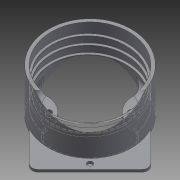
# Autodesk Inventor part: DiffuserCoupler
Saved by Autodesk Inventor 2014 SP2 (Build 180246200, 246)
## iProperties
Created: 2014-02-09
Part Number: DiffuserCoupler
Material: Generic
Document SubType Name: Modeling
Designer: jkao
Density: 1 g/cm^3
Appearance: Default
Author: jkao
Autodesk Inventor part; units mm, degrees
ref_plane "YZ Plane" through (0, 0, 0) normal (1, 0, 0) x (0, 1, 0)
ref_plane "XZ Plane" through (0, 0, 0) normal (0, 1, 0) x (-1, 0, 0)
ref_plane "XY Plane" through (0, 0, 0) normal (0, 0, 1) x (1, 0, 0)
sketch "Collar Profile" plane through (0, 0, 0) normal (0, 0, 1) x (1, 0, 0)
  circle A0 centre (0, 0) radius 13.75
  circle A1 centre (0, 0) radius 14.75
  dimension "collarInnerDiameter" = 27.5
  dimension "d74" = 29.5
  constraints: 2 centre point
  measures "collarInnerDiameter" diameter of A0
  measures "d74" diameter of A1
extrude "Collar" add sketch "Collar Profile" along normal blind 16
sketch "Thread Profile" plane through (0, 0, 0) normal (0, 1, 0) x (-1, 0, 0)
  line L0 (0, 27.549911) -> (0, -8)
  line L1 (13.75, 13) -> (13.15, 12.915052)
  line L2 (13.75, 13) -> (13.75, 12)
  line L3 (13.15, 12.915052) -> (13.15, 12.715052)
  line L4 (13.75, 12) -> (13.15, 12.715052)
  line L5 (13.75, 12) -> (14.386651, 12) construction
  line L6 (-14.75, 0) -> (14.75, 0)
  point P0 (0, 0)
  dimension "d98" = 1
  dimension "d99" = 130
  dimension "d100" = 12
  dimension "d125" = 0.2
  dimension "d127" = 0.6
  dimension "d128" = 13.75
  constraints: 12 end point, 2 vertical, 1 horizontal
  measures "d98" distance of L1.start L2.end
  measures "d99" angle of L5 L4
  measures "d100" distance between parallel lines of L5 L6
  measures "d125" distance of L1.end L3.end
  measures "d127" distance between parallel lines of L3 L2
  measures "d128" distance between parallel lines of L0 L2
coil "Diffuser Thread" sketch "Thread Profile" operation add axis through (0, 0, 27.549911) along (0, 0, -1) pitch 3 turns 2.5 hand right
fillet "Fillet3" radius 3 1 edges at (-13.15, 0, 12.8151)
sketch "Screw Tab Profile" plane through (0, 0, 0) normal (0, 0, -1) x (-1, 0, 0)
  circle A0 centre (0, 0) radius 13.75
  circle A1 centre (0, 0) radius 14.75
  arc A2 (-13.249986, -6.48077) -> (-13.249986, 6.48077) centre (-13.749609, 0) ccw
  arc A3 (13.249999, 6.480742) -> (13.249999, -6.480742) centre (13.749984, 0) ccw
  arc A4 (3.21587, 13.368645) -> (-3.215881, 13.368643) centre (-0.000006, 14.75) ccw
  arc A5 (-3.215876, -13.368644) -> (3.215876, -13.368644) centre (0, -14.75) ccw
  circle A6 centre (0, 0) radius 14.75
  line L0 (-13.75, 18.25) -> (13.75, 18.25)
  line L1 (13.75, 18.25) -> (13.75, -18.25)
  line L2 (13.75, -18.25) -> (-13.75, -18.25)
  line L3 (-13.75, -18.25) -> (-13.75, 18.25)
  point P0 (-9.249609, 0)
  point P1 (9.249984, 0)
  point P2 (-0.0003, 16.4)
  point P3 (0, -16.4)
  dimension "d103" = 6.5
  dimension "d105" = 6.5
  dimension "d106" = 3.5
  dimension "d108" = 4.5
  dimension "d109" = 4.5
  dimension "d121" = 3.5
  dimension "d122" = 1.65
  dimension "d123" = 1.65
  dimension "d129" = 29.5
  dimension "d133" = 36.5
  dimension "d134" = 27.5
  dimension "d135" = 13.75
  dimension "d136" = 13.75
  constraints: 17 point on circle, 8 end point, 5 centre point, 2 parallel, 1 horizontal, 1 perpendicular, 1 vertical alignment, 1 other
  measures "d103" radius of A2
  measures "d105" radius of A3
  measures "d106" radius of A4
  measures "d108" distance of A2.centre point (-9.25, 0)
  measures "d109" distance of A3.centre point (9.25, 0)
  measures "d122" distance of point (0, -16.4) A5.centre
  measures "d123" distance of A4.centre point (0, 16.4)
  measures "d129" diameter of A1
  measures "d133" distance between parallel lines of L2 L0
  measures "d134" distance between parallel lines of L1 L3
  measures "d135" distance from line of L3 A0.centre
  measures "d136" distance from line of L1 A0.centre
extrude "Tabs" add sketch "Screw Tab Profile" against normal blind 0.9 contours A0 A4 A1 | A3 A1 L1 A0 | A0 A3 | A4 L0 L1 A1 | A1 A4 | A2 A0 | A0 L3 A1 A2 | A1 L3 L0 A4 | L1 A1 A3 A0 | L1 A1 | A0 A2 A1 L3 | L3 A1 | L1 L2 A5 A1 | A5 A1 A0 | A1 A5 L2 L3 | A5 A1
hole "Screw Holes" at (9.249609, 0, 0) at (-9.249984, 0, 0) at (0.0003, 16.4, 0) at (0, -16.4, 0) direction (0, 0, 1) diameter 1.7 end through all clearance for "Socket Head Cap Screw" size "M1.6" standard "Ansi Metric M Profile"
fillet "Fillet4" radius 2 4 edges at (-13.75, -18.25, 0.45) (13.75, -18.25, 0.45) (-13.75, 18.25, 0.45) (13.75, 18.25, 0.45)
fillet "Fillet6" radius 2.5 7 edges at (13.3604, 3.25, 0.9) (13.3604, -3.25, 0.9) (-13.75, 0, 0.9) (-12.2136, -6.3158, 0.45) (-12.2136, 6.3158, 0.45) (12.2136, -6.3159, 0.45) (12.2136, 6.3159, 0.45)
equation "\"d128\" = 0.5 * collarInnerDiameter"
equation "\"d135\" = d136"
body "Solid3"
